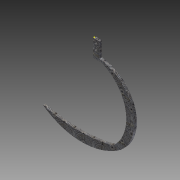
# Autodesk Inventor part: legplate
Saved by Autodesk Inventor 2015 (Build 190159000, 159)
## iProperties
Created: 2020-01-20
Part Number: legplate
Material: CFRP
Document SubType Name: Modeling
Designer: hp
Density: 1.43 g/cm^3
Appearance: Carbon Fiber
Author: hp
Autodesk Inventor part; units mm, degrees
ref_plane "YZ Plane" through (0, 0, 0) normal (1, 0, 0) x (0, 1, 0)
ref_plane "XZ Plane" through (0, 0, 0) normal (0, 1, 0) x (-1, 0, 0)
ref_plane "XY Plane" through (0, 0, 0) normal (0, 0, 1) x (1, 0, 0)
sketch "Sketch1" plane through (0, 0, 0) normal (1, 0, 0) x (0, 1, 0)
  line L0 (18.6276, 30.145) -> (-681.3735, 30.145)
  line L1 (18.6276, 30.145) -> (18.6276, -29.8549)
  line L2 (18.6276, -29.8549) -> (-681.3735, -29.8549)
  line L3 (-681.3735, 30.145) -> (-1317.975, 30.145)
  line L4 (-1317.975, 30.145) -> (-1300.7166, -29.8549)
  line L5 (-1300.7166, -29.8549) -> (-681.3735, -29.8549)
  point P0 (0, 0)
  dimension "d0" = 700.0011
  dimension "d1" = 59.9999
  constraints: 12 end point, 3 horizontal, 1 parallel, 1 vertical
  measures "d0" distance of L0.start L0.end
  measures "d1" distance of L0.start L1.end
extrude "Extrusion1" add sketch "Sketch1" along normal blind 150
sketch "Sketch2" plane through (0, 18.6276, 30.145) normal (0, 1, 0) x (1, 0, 0)
  line L0 (30.0948, 48.0392) -> (130.9532, 48.0392) construction
  line L1 (130.9532, 48.0392) -> (130.9532, 12.2508) construction
  line L2 (130.9532, 12.2508) -> (30.0948, 12.2508) construction
  line L3 (30.0948, 12.2508) -> (30.0948, 48.0392) construction
  point P0 (0, 30.145)
  constraints: 2 other
fillet "Fillet1" [suppressed]
chamfer "Chamfer1" [suppressed]
sketch "Sketch3" plane through (150, 18.6276, -29.8549) normal (0, 0, -1) x (-1, 0, 0)
  circle A0 centre (86.2337, -73.5365) radius 25.4
  circle A1 centre (86.2337, -207.3813) radius 25.4
  point P0 (150, -18.6276)
  dimension "d8" = 50.8
  dimension "d9" = 50.8
  constraints: 2 centre point
  measures "d8" diameter of A0
  measures "d9" diameter of A1
extrude "Extrusion2" cut sketch "Sketch3" against normal blind 150
fillet "Fillet2" radius 203.2 1 edges at (150, -1309.3458, 0.1451)
sketch "Sketch4" plane through (0, 18.6276, 30.145) normal (0, 0, 1) x (1, 0, 0)
  line L0 (0, 0) -> (0, -1336.6026) projected
  line L1 (0, -407.0419) -> (196.678, -407.0419)
  line L2 (196.678, -407.0419) -> (196.678, -1363.7468)
  line L3 (196.678, -1363.7468) -> (0, -1363.7468)
  line L4 (0, -1363.7468) -> (0, -407.0419)
  point P0 (0, -18.6276)
  constraints: 8 end point, 2 parallel, 1 horizontal, 1 perpendicular, 1 point on line
extrude "Extrusion3" cut sketch "Sketch4" against normal blind 76.2
sketch "Sketch5" plane through (0, 18.6276, 30.145) normal (0, 0, 1) x (1, 0, 0)
  arc A0 (657.8206, -1984.0725) -> (111.0415, -352.1801) centre (55.7755, -1278.2451) ccw
  arc A1 (-1190.1731, -1984.0725) -> (664.0722, -1978.692) centre (-266.7148, -718.5694) ccw
  arc A2 (473.6908, -1984.0725) -> (0.5095, -352.1801) centre (-147.8493, -1279.7458) ccw
  arc A3 (-1190.1731, -1984.0725) -> (473.6908, -1984.0725) centre (-358.2411, 1144.2439) ccw
  line L0 (0.5095, -352.1801) -> (111.0415, -352.1801)
  line L1 (150, -407.0419) -> (150, 0) projected
  line L2 (150, 0) -> (150, -407.0419) projected
  line L3 (150, -355.3299) -> (150, -388.8618)
  point P0 (0, -18.6276)
  constraints: 11 point on circle, 4 centre point, 4 end point, 2 point on line, 1 perpendicular
extrude "Extrusion4" add sketch "Sketch5" against normal blind 60.0024 contours A1 A3 A2 L1 A0
body "Solid1"
